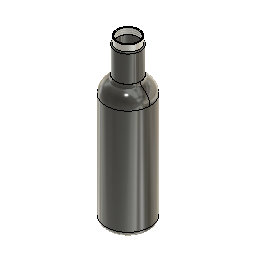
Bottle v1 (Autodesk Fusion 360 design; units mm, degrees)
Autodesk Fusion 360 part; units mm, degrees
sketch "Sketch1" plane through (0, 0, 0) normal (0, 0, 1) x (1, 0, 0)
  circle A0 centre (0, 0) radius 40
  dimension "d1" = 80
  constraint coincident A0.centre origin
  measures "d1" diameter of A0
extrude "Extrude1" add sketch "Sketch1" along normal blind 198 from surface at 4 thin wall 4 inside makes body 1
sketch "Sketch4" plane through (0, 0, 0) normal (0, 1, 0) x (1, 0, 0)
  line L0 (-40, -202) -> (40, -202)
  line L1 (0, -202) -> (22.5, -202)
  line L2 (22.5, -202) -> (22.5, -232) construction
  spline S0 degree 5 poles (40, -202) (40, -202.9025) (39.9213, -204.6712) (39.5674, -207.2148) (38.6477, -210.3815) (36.8981, -213.931) (34.7489, -217.0279) (32.4263, -219.6309) (30.1545, -221.7136) (28.1291, -223.2786) (26.4896, -224.3732) (25.2889, -225.1091) (24.4662, -225.678) (23.9063, -226.2943) (23.4868, -227.147) (23.1324, -228.3422) (22.8716, -229.6079) (22.6831, -230.7352) (22.5605, -231.5653) (22.5, -232) knots 0 0 0 0 0 0 0.066667 0.133333 0.2 0.266667 0.333333 0.4 0.466667 0.533333 0.6 0.666667 0.733333 0.8 0.866667 0.933333 1 1 1 1 1 1
  line L3 (40, -196.8948) -> (40, -207.1052)
  spline S1 degree 3 poles (36, -202) (36, -205.1073) (35.3291, -207.7737) (34.1881, -210.1958) (32.7221, -213.308) (30.4626, -215.9522) (28.4177, -217.8333) (27.1053, -219.0406) (25.9099, -219.925) (24.9581, -220.5712) (24.0837, -221.1648) (23.418, -221.5412) (22.637, -222.0992) (22.1114, -222.4746) (21.5, -222.9822) (20.9778, -223.6354) (20.417, -224.3368) (20.0218, -225.1229) (19.7453, -225.8614) (19.3143, -227.0128) (19.0742, -228.1547) (18.8325, -229.5481) (18.73, -230.139) (18.6325, -230.7708) (18.5382, -231.4485) knots 0 0 0 0 0.162876 0.162876 0.162876 0.372157 0.372157 0.372157 0.506468 0.506468 0.506468 0.629851 0.629851 0.629851 0.71287 0.71287 0.71287 0.80203 0.80203 0.80203 0.941048 0.941048 0.941048 1 1 1 1
  line L4 (22.5, -232) -> (18.5382, -232)
  line L5 (18.5382, -232) -> (18.5382, -231.4485)
  point P0 (0, -202)
  point P1 (26.7396, -224.1916)
  point P2 (23.8928, -226.4283)
  dimension "d9" = 22.5
  dimension "d10" = 30
  dimension "d25" = 4
  constraint coincident P0 L0
  constraint midpoint P0 L0
  constraint coincident P0 L1.start
  constraint parallel L0 L1
  constraint perpendicular L0 L2
  constraint coincident L0.end S0.start
  constraint midpoint L0.end L3
  constraint perpendicular L2 L4
  constraint perpendicular L4 L5
  measures "d9" distance of P0 L1.end
  measures "d10" distance of L1.end L2.end
revolve "Revolve1" add sketch "Sketch4" angle 360 about axis through (0, 0, 1.75) along (0, 0, 1) bodies 1
extrude "Extrude4" add 1 faces at (20.7819, -3.2737, 232) along direction (0, 0, 1) blind 50 on bodies 1 bodies 1
extrude "Extrude5" add sketch "Sketch1" along normal blind 4 bodies 1
fillet "Fillet3" radius 10 2 edges at (-37.2931, -14.4646, 0) (-33.5638, -13.0182, 4) on bodies 1
fillet "Fillet4" radius 2 2 edges at (-20.9774, -8.1363, 232) (-17.2837, -6.7037, 231.4485) on bodies 1
fillet "Fillet5" radius 2 1 edges at (-20.9774, -8.1363, 282) on bodies 1
extrude "Extrude6" add 1 faces at (19.7697, -1.0185, 282) along direction (0, 0, 1) blind 12 separate body on bodies 1 makes body 2
fillet "Fillet6" radius 0.75 1 faces at (19.7697, -1.0185, 294) on bodies 2
thread "Thread1" "ANSI Unified Screw Threads 1.5625 1 9/16-8 UN 3B" major diameter 39.6875 minor diameter 36.4388 pitch 3.175 angle 60 resizes the face on face at (18.5152, -0.9241, 289.5) on bodies 2
